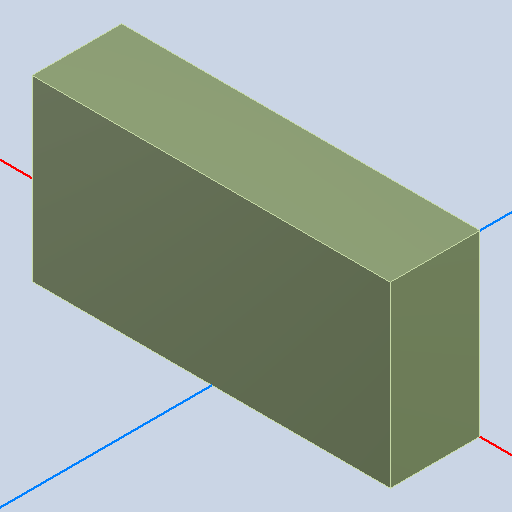
# Autodesk Inventor part: M0805
Saved by Autodesk Inventor 2022 (Build 260153000, 153)
## iProperties
Created: 2022-12-23
Part Number: M0805
Material: Типовые
Document SubType Name: Modeling
Designer: Ivan Petrov
Density: 1 g/cm^3
Appearance: M0805, M0805
Author: Ivan Petrov
Autodesk Inventor part; units mm, degrees
ref_plane "YZ Plane" through (0, 0, 0) normal (1, 0, 0) x (0, 1, 0)
ref_plane "XZ Plane" through (0, 0, 0) normal (0, 1, 0) x (-1, 0, 0)
ref_plane "XY Plane" through (0, 0, 0) normal (0, 0, 1) x (1, 0, 0)
sketch "M0805, M0805_1" plane through (0, 0, 0) normal (0, 0, 1) x (1, 0, 0)
  line L0 (-1.9984, 1.0084) -> (1.9984, 1.0084)
  line L1 (1.9984, 1.0084) -> (1.9984, -0.983)
  line L2 (1.9984, -0.983) -> (-1.9984, -0.983)
  line L3 (-1.9984, -0.983) -> (-1.9984, 1.0084)
  constraints: 8 end point
extrude "Выдавливание1" add sketch "M0805, M0805_1" along normal blind 1
